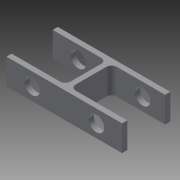
# Autodesk Inventor part: Slider ver2
Saved by Autodesk Inventor 2015 (Build 190159000, 159)
## iProperties
Created: 2016-05-27
Part Number: Slider ver2
Material: Generic
Document SubType Name: Modeling
Designer: Toby
Density: 1 g/cm^3
Appearance: Default
Author: Toby
Autodesk Inventor part; units mm, degrees
ref_plane "YZ Plane" through (0, 0, 0) normal (1, 0, 0) x (0, 1, 0)
ref_plane "XZ Plane" through (0, 0, 0) normal (0, 1, 0) x (-1, 0, 0)
ref_plane "XY Plane" through (0, 0, 0) normal (0, 0, 1) x (1, 0, 0)
sketch "Sketch1" plane through (0, 0, 0) normal (0, 0, 1) x (1, 0, 0)
  line L0 (-5.3333, 0.9286) -> (39.6667, 0.9286)
  line L1 (39.6667, 0.9286) -> (39.6667, -1.0714)
  line L2 (39.6667, -1.0714) -> (-5.3333, -1.0714)
  line L3 (-5.3333, -1.0714) -> (-5.3333, 0.9286)
  line L4 (-5.3333, 18.9286) -> (38.4017, 18.9286)
  line L5 (38.4017, 18.9286) -> (38.4017, 16.9286)
  line L6 (38.4017, 16.9286) -> (-5.3333, 16.9286)
  line L7 (-5.3333, 16.9286) -> (-5.3333, 18.9286)
  line L8 (16.5342, 16.9286) -> (15.5342, 16.9286)
  line L9 (15.5342, 16.9286) -> (15.5342, 0.9286)
  line L10 (15.5342, 0.9286) -> (16.5342, 0.9286)
  line L11 (16.5342, 0.9286) -> (16.5342, 16.9286)
  line L12 (16.5342, 16.9286) -> (17.5342, 16.9286)
  line L13 (17.5342, 16.9286) -> (17.5342, 0.9286)
  line L14 (17.5342, 0.9286) -> (16.5342, 0.9286)
  line L15 (16.5342, 0.9286) -> (16.5342, 16.9286)
  point P0 (0, 0)
  dimension "d0" = 2
  dimension "d1" = 45
  dimension "d2" = 2
  dimension "d3" = 1
  dimension "d4" = 1
  dimension "d5" = 20
  constraints: 32 end point, 8 parallel, 4 horizontal, 4 perpendicular, 2 point on line, 1 midpoint
  measures "d0" distance of L2.end L0.start
  measures "d1" distance of L0.start L0.end
  measures "d2" distance of L6.end L4.start
  measures "d3" distance between parallel lines of L9 L11
  measures "d4" distance between parallel lines of L15 L13
  measures "d5" distance between parallel lines of L2 L4
extrude "Extrusion1" add sketch "Sketch1" along normal blind 10
sketch "Sketch2" plane through (-5.3333, 18.9286, 0) normal (0, 1, 0) x (1, 0, 0)
  circle A0 centre (10, -5) radius 3
  circle A1 centre (35, -5) radius 3
  line L0 (0, 0) -> (0, -10) projected
  line L1 (45, 0) -> (45, -10) projected
  line L2 (43.735, 0) -> (0, 0) projected
  point P0 (5.3333, 0)
  dimension "d8" = 6
  dimension "d9" = 6
  dimension "d10" = 10
  dimension "d11" = 10
  dimension "d12" = 5
  dimension "d13" = 5
  constraints: 2 centre point
  measures "d8" diameter of A0
  measures "d9" diameter of A1
  measures "d10" distance from line of L0 A0.centre
  measures "d11" distance from line of L1 A1.centre
  measures "d12" distance from line of L2 A0.centre
  measures "d13" distance from line of L2 A1.centre
extrude "Extrusion2" cut sketch "Sketch2" against normal blind 20
fillet "Fillet1" radius 2 4 edges at (17.5342, 0.9286, 5) (15.5342, 0.9286, 5) (17.5342, 16.9286, 5) (15.5342, 16.9286, 5)
body "Solid1"
